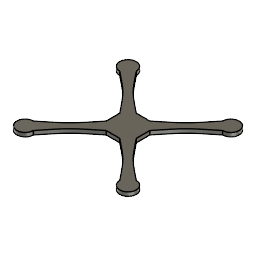
Drone 4 Polegadas (Autodesk Fusion 360 design; units mm, degrees)
Autodesk Fusion 360 part; units mm, degrees
sketch "Esboço1" plane through (0, 0, 0) normal (0, 0, 1) x (1, 0, 0)
  circle A0 centre (-65.8, 65.8) radius 10.65
  circle A1 centre (65.8, 65.8) radius 10.65
  circle A2 centre (-65.8, -65.8) radius 10.65
  circle A3 centre (65.8, -65.8) radius 10.65
  line L0 (-65.8, 65.8) -> (-19.2724, 19.2724) construction
  line L1 (0, 65.8) -> (0, -65.8) construction
  line L2 (-65.8, 0) -> (65.8, 0) construction
  line L3 (65.8, 65.8) -> (19.2724, 19.2724) construction
  line L4 (-65.8, -65.8) -> (-19.2724, -19.2724) construction
  line L5 (65.8, -65.8) -> (19.2724, -19.2724) construction
  line L6 (13.2724, -19.2724) -> (-13.2724, -19.2724)
  line L7 (-19.2724, -13.2724) -> (-19.2724, 13.2724)
  line L8 (-13.2724, 19.2724) -> (13.2724, 19.2724)
  line L9 (19.2724, 13.2724) -> (19.2724, -13.2724)
  line L10 (19.2724, -19.2724) -> (-19.2724, 19.2724) construction
  line L11 (-19.2724, -19.2724) -> (19.2724, 19.2724) construction
  line L12 (-42.5362, 31.8862) -> (-37.2112, 37.2112) construction
  line L13 (-31.8862, 42.5362) -> (-37.2112, 37.2112) construction
  spline S0 degree 2 poles (-65.8, 55.15) (-39.8737, 34.5487) (-19.2724, 8.6224) knots 0 0 0 6.604196 6.604196 6.604196 weights 1 3 1
  spline S1 degree 2 poles (-55.15, 65.8) (-34.5487, 39.8737) (-8.6224, 19.2724) knots 0 0 0 6.604196 6.604196 6.604196 weights 1 3 1
  arc A4 (-13.2724, 19.2724) -> (-19.2724, 13.2724) centre (-13.2724, 13.2724) ccw
  arc A5 (19.2724, 13.2724) -> (13.2724, 19.2724) centre (13.2724, 13.2724) ccw
  arc A6 (-19.2724, -13.2724) -> (-13.2724, -19.2724) centre (-13.2724, -13.2724) ccw
  arc A7 (13.2724, -19.2724) -> (19.2724, -13.2724) centre (13.2724, -13.2724) ccw
  spline S2 degree 2 poles (65.8, 55.15) (39.8737, 34.5487) (19.2724, 8.6224) knots 0 0 0 6.604196 6.604196 6.604196 weights 1 3 1
  spline S3 degree 2 poles (55.15, 65.8) (34.5487, 39.8737) (8.6224, 19.2724) knots 0 0 0 6.604196 6.604196 6.604196 weights 1 3 1
  spline S4 degree 2 poles (-65.8, -55.15) (-39.8737, -34.5487) (-19.2724, -8.6224) knots 0 0 0 6.604196 6.604196 6.604196 weights 1 3 1
  spline S5 degree 2 poles (-55.15, -65.8) (-34.5487, -39.8737) (-8.6224, -19.2724) knots 0 0 0 6.604196 6.604196 6.604196 weights 1 3 1
  spline S6 degree 2 poles (55.15, -65.8) (34.5487, -39.8737) (8.6224, -19.2724) knots 0 0 0 6.604196 6.604196 6.604196 weights 1 3 1
  spline S7 degree 2 poles (65.8, -55.15) (39.8737, -34.5487) (19.2724, -8.6224) knots 0 0 0 6.604196 6.604196 6.604196 weights 1 3 1
  dimension "d1" = 131.6
  dimension "d2" = 131.6
  dimension "d3" = 21.3
  dimension "d4" = 21.3
  dimension "d5" = 21.3
  dimension "d6" = 21.3
  dimension "d7" = 65.8
  dimension "d10" = 6
  constraint coincident A0.centre L0.start
  constraint symmetric A0.centre L1 A1.centre
  constraint symmetric L0.end L1 L3.end
  constraint symmetric A0.centre L2 A2.centre
  constraint symmetric L0.end L2 L4.end
  constraint symmetric L2 A1.centre A3.centre
  constraint symmetric L2 L3.end L5.end
  constraint horizontal L6
  constraint perpendicular L6 L7
  constraint parallel L6 L8
  constraint parallel L7 L9
  constraint coincident L10 origin
  constraint coincident L11 origin
  constraint coincident A0 S0.start
  constraint coincident L7 S0.end
  constraint coincident A0 S1.start
  constraint coincident L8 S1.end
  constraint coincident L0 L12.end
  constraint perpendicular L0 L12
  constraint perpendicular L0 L13
  constraint coincident L0.end L8
  constraint coincident L0.end L7
  constraint tangent L8 A4
  constraint tangent L7 A4
  constraint coincident L3.end L8
  constraint coincident L3.end L9
  constraint tangent L8 A5
  constraint tangent L9 A5
  constraint equal A4 A5
  constraint coincident L4.end L6
  constraint coincident L4.end L7
  constraint tangent L6 A6
  constraint tangent L7 A6
  constraint equal A4 A6
  constraint coincident L5.end L9
  constraint coincident L5.end L6
  constraint tangent L9 A7
  constraint tangent L6 A7
  constraint equal A4 A7
  constraint symmetric L1 S0.start S2.start
  constraint symmetric L1 S0.end S2.end
  constraint symmetric L1 S1.start S3.start
  constraint symmetric L1 S1.end S3.end
  constraint symmetric L1 S0 S2
  constraint symmetric L1 S1 S3
  constraint symmetric L2 S0.start S4.start
  constraint symmetric L2 S0.end S4.end
  constraint symmetric L2 S1.start S5.start
  constraint symmetric L2 S1.end S5.end
  constraint symmetric L2 S0 S4
  constraint symmetric L2 S1 S5
  constraint symmetric L2 S2.start S7.start
  constraint symmetric L2 S2.end S7.end
  constraint symmetric L2 S2 S7
  constraint symmetric L2 S3.start S6.start
  constraint symmetric L2 S3.end S6.end
  constraint symmetric L2 S3 S6
  measures "d1" distance of A0.centre A1.centre
  measures "d2" distance of A0.centre A2.centre
  measures "d3" diameter of A0
  measures "d4" diameter of A1
  measures "d5" diameter of A2
  measures "d6" diameter of A3
  measures "d7" distance of A0.centre L0.end
  measures "d10" radius of A4
extrude "Extrusão1" add sketch "Esboço1" along normal blind 5
equation "d8 = 0.75"
equation "d9 = 0.75"
equation "d11 = d8"
equation "d12 = d9"
equation "d13 = d8"
equation "d14 = d9"
equation "d15 = d12"
equation "d16 = d11"
